Autodesk Inventor part; units mm, degrees
(part 2 of 2)
sketch "Sketch4" plane through (0, 0, 0) normal (0, -1, 0) x (1, 0, 0)
  circle A0 centre (-88.9635, -7.901) radius 1.7 projected
  circle A1 centre (-21.7635, -7.9073) radius 1.7 projected
  circle A2 centre (-22.0668, -135.0168) radius 1.7 projected
  circle A3 centre (-57.3517, -134.2073) radius 1.7 projected
  circle A4 centre (-128.0635, -215.5073) radius 1.7 projected
  circle A5 centre (-1.6635, -245.9073) radius 1.7 projected
  circle A6 centre (-19.8635, -215.5073) radius 1.7 projected
  circle A7 centre (-1.6635, -21.6073) radius 1.7 projected
  circle A8 centre (-16.4635, -2.0899) radius 1.7 projected
  circle A9 centre (-128.0635, -2.0899) radius 1.7 projected
  line L0 (-3.3635, -123.4758) -> (0.2365, -123.4758) projected
  line L1 (0.2365, -123.4758) -> (0.2365, -129.7758) projected
  line L2 (0.2365, -129.7758) -> (-3.3635, -129.7758) projected
  line L3 (-3.3635, -129.7758) -> (-3.3635, -123.4758) projected
  line L4 (-30.1635, -0.1899) -> (-23.9635, -0.1899) projected
  line L5 (-23.9635, -0.1899) -> (-23.9635, -3.7899) projected
  line L6 (-23.9635, -3.7899) -> (-30.1635, -3.7899) projected
  line L7 (-30.1635, -3.7899) -> (-30.1635, -0.1899) projected
  line L8 (-33.5635, -213.6073) -> (-27.3634, -213.6073) projected
  line L9 (-27.3634, -213.6073) -> (-27.3634, -217.2073) projected
  line L10 (-27.3634, -217.2073) -> (-33.5635, -217.2073) projected
  line L11 (-33.5635, -217.2073) -> (-33.5635, -213.6073) projected
  line L12 (-141.7635, -0.1899) -> (-135.5635, -0.1899) projected
  line L13 (-135.5635, -0.1899) -> (-135.5635, -3.7899) projected
  line L14 (-135.5635, -3.7899) -> (-141.7635, -3.7899) projected
  line L15 (-141.7635, -3.7899) -> (-141.7635, -0.1899) projected
  line L16 (-141.7635, -213.6073) -> (-135.5635, -213.6073) projected
  line L17 (-135.5635, -213.6073) -> (-135.5635, -217.2073) projected
  line L18 (-135.5635, -217.2073) -> (-141.7635, -217.2073) projected
  line L19 (-141.7635, -217.2073) -> (-141.7635, -213.6073) projected
  line L20 (-3.3635, -29.1073) -> (0.2365, -29.1073) projected
  line L21 (0.2365, -29.1073) -> (0.2365, -35.3073) projected
  line L22 (0.2365, -35.3073) -> (-3.3635, -35.3073) projected
  line L23 (-3.3635, -35.3073) -> (-3.3635, -29.1073) projected
  line L24 (-3.3635, -253.4073) -> (0.2365, -253.4073) projected
  line L25 (0.2365, -253.4073) -> (0.2365, -259.6074) projected
  line L26 (0.2365, -259.6074) -> (-3.3635, -259.6074) projected
  line L27 (-3.3635, -259.6074) -> (-3.3635, -253.4073) projected
  line L28 (-120.5635, -0.1899) -> (-114.3635, -0.1899) projected
  line L29 (-114.3635, -0.1899) -> (-114.3635, -3.7899) projected
  line L30 (-114.3635, -3.7899) -> (-120.5635, -3.7899) projected
  line L31 (-120.5635, -3.7899) -> (-120.5635, -0.1899) projected
  line L32 (-120.5635, -213.6073) -> (-114.3635, -213.6073) projected
  line L33 (-114.3635, -213.6073) -> (-114.3635, -217.2073) projected
  line L34 (-114.3635, -217.2073) -> (-120.5635, -217.2073) projected
  line L35 (-120.5635, -217.2073) -> (-120.5635, -213.6073) projected
  line L36 (-3.3635, -232.2073) -> (0.2365, -232.2073) projected
  line L37 (0.2365, -232.2073) -> (0.2365, -238.4073) projected
  line L38 (0.2365, -238.4073) -> (-3.3635, -238.4073) projected
  line L39 (-3.3635, -238.4073) -> (-3.3635, -232.2073) projected
  line L40 (-8.9635, -0.1899) -> (-2.7635, -0.1899) projected
  line L41 (-2.7635, -0.1899) -> (-2.7635, -3.7899) projected
  line L42 (-2.7635, -3.7899) -> (-8.9635, -3.7899) projected
  line L43 (-8.9635, -3.7899) -> (-8.9635, -0.1899) projected
  line L44 (-3.3635, -7.9073) -> (0.2365, -7.9073) projected
  line L45 (0.2365, -7.9073) -> (0.2365, -14.1073) projected
  line L46 (0.2365, -14.1073) -> (-3.3635, -14.1073) projected
  line L47 (-3.3635, -14.1073) -> (-3.3635, -7.9073) projected
  line L48 (-12.3635, -213.6073) -> (-6.1635, -213.6073) projected
  line L49 (-6.1635, -213.6073) -> (-6.1635, -217.2073) projected
  line L50 (-6.1635, -217.2073) -> (-12.3635, -217.2073) projected
  line L51 (-12.3635, -217.2073) -> (-12.3635, -213.6073) projected
  line L52 (-194.5059, -23.9073) -> (-194.4204, -23.2582) projected
  line L53 (-194.4204, -23.2582) -> (-194.1699, -22.6533) projected
  line L54 (-194.1699, -22.6533) -> (-193.7713, -22.1339) projected
  line L55 (-193.7713, -22.1339) -> (-193.2519, -21.7353) projected
  line L56 (-193.2519, -21.7353) -> (-192.647, -21.4848) projected
  line L57 (-192.647, -21.4848) -> (-191.9979, -21.3993) projected
  line L58 (-191.9979, -21.3993) -> (-191.3488, -21.4848) projected
  line L59 (-191.3488, -21.4848) -> (-190.7439, -21.7353) projected
  line L60 (-190.7439, -21.7353) -> (-190.2245, -22.1339) projected
  line L61 (-190.2245, -22.1339) -> (-189.8259, -22.6533) projected
  line L62 (-189.8259, -22.6533) -> (-189.5754, -23.2582) projected
  line L63 (-189.5754, -23.2582) -> (-189.4899, -23.9073) projected
  line L64 (-189.4899, -23.9073) -> (-189.5754, -24.5564) projected
  line L65 (-189.5754, -24.5564) -> (-189.8259, -25.1613) projected
  line L66 (-189.8259, -25.1613) -> (-190.2245, -25.6807) projected
  line L67 (-190.2245, -25.6807) -> (-190.7439, -26.0793) projected
  line L68 (-190.7439, -26.0793) -> (-191.3488, -26.3299) projected
  line L69 (-191.3488, -26.3299) -> (-191.9979, -26.4153) projected
  line L70 (-191.9979, -26.4153) -> (-192.647, -26.3299) projected
  line L71 (-192.647, -26.3299) -> (-193.2519, -26.0793) projected
  line L72 (-193.2519, -26.0793) -> (-193.7713, -25.6807) projected
  line L73 (-193.7713, -25.6807) -> (-194.1699, -25.1613) projected
  line L74 (-194.1699, -25.1613) -> (-194.4204, -24.5564) projected
  line L75 (-194.4204, -24.5564) -> (-194.5059, -23.9073) projected
  line L76 (-14.004, -16.4042) -> (-13.929, -15.8348) projected
  line L77 (-13.929, -15.8348) -> (-13.7092, -15.3042) projected
  line L78 (-13.7092, -15.3042) -> (-13.3596, -14.8486) projected
  line L79 (-13.3596, -14.8486) -> (-12.904, -14.499) projected
  line L80 (-12.904, -14.499) -> (-12.3734, -14.2792) projected
  line L81 (-12.3734, -14.2792) -> (-11.804, -14.2042) projected
  line L82 (-11.804, -14.2042) -> (-11.2346, -14.2792) projected
  line L83 (-11.2346, -14.2792) -> (-10.704, -14.499) projected
  line L84 (-10.704, -14.499) -> (-10.2483, -14.8486) projected
  line L85 (-10.2483, -14.8486) -> (-9.8987, -15.3042) projected
  line L86 (-9.8987, -15.3042) -> (-9.679, -15.8348) projected
  line L87 (-9.679, -15.8348) -> (-9.604, -16.4042) projected
  line L88 (-9.604, -16.4042) -> (-9.679, -16.9736) projected
  line L89 (-9.679, -16.9736) -> (-9.8987, -17.5042) projected
  line L90 (-9.8987, -17.5042) -> (-10.2483, -17.9599) projected
  line L91 (-10.2483, -17.9599) -> (-10.704, -18.3095) projected
  line L92 (-10.704, -18.3095) -> (-11.2346, -18.5293) projected
  line L93 (-11.2346, -18.5293) -> (-11.804, -18.6042) projected
  line L94 (-11.804, -18.6042) -> (-12.3734, -18.5293) projected
  line L95 (-12.3734, -18.5293) -> (-12.904, -18.3095) projected
  line L96 (-12.904, -18.3095) -> (-13.3596, -17.9599) projected
  line L97 (-13.3596, -17.9599) -> (-13.7092, -17.5042) projected
  line L98 (-13.7092, -17.5042) -> (-13.929, -16.9736) projected
  line L99 (-13.929, -16.9736) -> (-14.004, -16.4042) projected
  line L100 (-21.9351, -237.6571) -> (-21.8831, -237.0851) projected
  line L101 (-21.8831, -237.0851) -> (-21.685, -236.5461) projected
  line L102 (-21.685, -236.5461) -> (-21.354, -236.0767) projected
  line L103 (-21.354, -236.0767) -> (-20.9129, -235.7089) projected
  line L104 (-20.9129, -235.7089) -> (-20.3916, -235.4679) projected
  line L105 (-20.3916, -235.4679) -> (-19.8257, -235.37) projected
  line L106 (-19.8257, -235.37) -> (-19.2537, -235.4219) projected
  line L107 (-19.2537, -235.4219) -> (-18.7147, -235.6201) projected
  line L108 (-18.7147, -235.6201) -> (-18.2453, -235.951) projected
  line L109 (-18.2453, -235.951) -> (-17.8776, -236.3922) projected
  line L110 (-17.8776, -236.3922) -> (-17.6365, -236.9134) projected
  line L111 (-17.6365, -236.9134) -> (-17.5386, -237.4793) projected
  line L112 (-17.5386, -237.4793) -> (-17.5905, -238.0513) projected
  line L113 (-17.5905, -238.0513) -> (-17.7887, -238.5903) projected
  line L114 (-17.7887, -238.5903) -> (-18.1196, -239.0597) projected
  line L115 (-18.1196, -239.0597) -> (-18.5608, -239.4274) projected
  line L116 (-18.5608, -239.4274) -> (-19.0821, -239.6685) projected
  line L117 (-19.0821, -239.6685) -> (-19.648, -239.7664) projected
  line L118 (-19.648, -239.7664) -> (-20.22, -239.7145) projected
  line L119 (-20.22, -239.7145) -> (-20.759, -239.5163) projected
  line L120 (-20.759, -239.5163) -> (-21.2284, -239.1854) projected
  line L121 (-21.2284, -239.1854) -> (-21.5961, -238.7443) projected
  line L122 (-21.5961, -238.7443) -> (-21.8371, -238.223) projected
  line L123 (-21.8371, -238.223) -> (-21.9351, -237.6571) projected
  line L124 (2.2365, 1.8101) -> (2.2365, -264.9073) projected
  line L125 (-206.7635, 1.8101) -> (2.2365, 1.8101) projected
  line L126 (-206.7635, -264.9073) -> (-206.7635, 1.8101) projected
  line L127 (2.2365, -264.9073) -> (-206.7635, -264.9073) projected
  circle A10 centre (-11.804, -16.4042) radius 2.1812
  circle A11 centre (-19.7368, -237.5682) radius 2.1812
  point P0 (0, 0)
  constraints: 6 tangent, 2 centre point
hole "Hole3" at (-19.7368, 0, -237.5682) at (-11.804, 0, -16.4042) direction (0, 1, 0) diameter 4.5 end through all
sketch "Sketch5" plane through (0, 3, 0) normal (0, 1, 0) x (1, 0, 0)
  line L0 (-189.5754, 23.2582) -> (-189.8259, 22.6533) projected
  line L1 (-192.647, 21.4848) -> (-193.2519, 21.7353) projected
  line L2 (-191.9979, 26.4153) -> (-191.3488, 26.3299) projected
  circle A0 centre (-191.9979, 23.9073) radius 2.4865
  point P0 (0, 0)
  constraints: 3 tangent, 1 centre point
hole "Hole4" at (-191.9979, 3, -23.9073) direction (0, -1, 0) diameter 5.2 end through all
body "Solid1"
